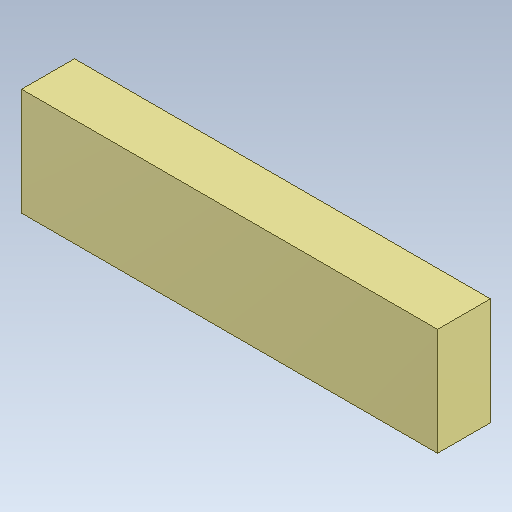
# Autodesk Inventor part: 3V
Saved by Autodesk Inventor 2021 (Build 250183000, 183)
## iProperties
Created: 2020-11-18
Part Number: 3V
Material: Generic
Document SubType Name: Modeling
Designer: Admin
Density: 1 g/cm^3
Appearance: DO35-7, 3V
Author: Admin
Autodesk Inventor part; units mm, degrees
ref_plane "YZ Plane" through (0, 0, 0) normal (1, 0, 0) x (0, 1, 0)
ref_plane "XZ Plane" through (0, 0, 0) normal (0, 1, 0) x (-1, 0, 0)
ref_plane "XY Plane" through (0, 0, 0) normal (0, 0, 1) x (1, 0, 0)
sketch "DO35-7, 3V_16" plane through (0, 0, 0) normal (0, 0, 1) x (1, 0, 0)
  line L0 (-3.81, 1.016) -> (4.064, 1.016)
  line L1 (4.064, 1.016) -> (4.064, -1.016)
  line L2 (4.064, -1.016) -> (-3.81, -1.016)
  line L3 (-3.81, -1.016) -> (-3.81, 1.016)
  constraints: 8 end point
extrude "Extrusion1" add sketch "DO35-7, 3V_16" along normal blind 1
body "Solid1"
